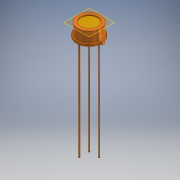
# Autodesk Inventor part: Thorlabs_FDS010
Saved by Autodesk Inventor 2018 (Build 220112000, 112)
## iProperties
Created: 2017-06-15
Part Number: Thorlabs_FDS010
Material: Gold
Document SubType Name: Modeling
Designer: yhlien
Density: 19.3 g/cm^3
Appearance: Metal 1600F Hot
Author: yhlien
Autodesk Inventor part; units mm, degrees
ref_plane "YZ Plane" through (0, 0, 0) normal (1, 0, 0) x (0, 1, 0)
ref_plane "XZ Plane" through (0, 0, 0) normal (0, 1, 0) x (-1, 0, 0)
ref_plane "XY Plane" through (0, 0, 0) normal (0, 0, 1) x (1, 0, 0)
sketch "Sketch1" plane through (0, 0, 0) normal (0, 0, 1) x (1, 0, 0)
  circle A0 centre (0, 0) radius 4.55
  dimension "d0" = 9.1
  constraints: 1 centre point, 1 coincident
  measures "d0" diameter of A0
extrude "Base" add sketch "Sketch1" along normal blind 0.71
sketch "Sketch2" plane through (0, 0, 0.71) normal (0, 0, 1) x (1, 0, 0)
  circle A0 centre (0, 0) radius 4.15
  dimension "d3" = 8.3
  constraints: 1 centre point, 1 coincident
  measures "d3" diameter of A0
extrude "Can: Outer Wall" add sketch "Sketch2" along normal blind 3.9
sketch "Sketch3" plane through (0, 0, 4.61) normal (0, 0, 1) x (1, 0, 0)
  circle A0 centre (0, 0) radius 3.85
  dimension "d6" = 7.7
  constraints: 1 centre point, 1 coincident
  measures "d6" diameter of A0
extrude "Can: Inner Wall" cut sketch "Sketch3" against normal blind 3.9
sketch "Sketch4" plane through (0, 0, 4.61) normal (0, 0, 1) x (1, 0, 0)
  circle A0 centre (0, 0) radius 3.85
  dimension "d9" = 7.7
  constraints: 1 centre point, 1 coincident
  measures "d9" diameter of A0
extrude "Can: Top" add sketch "Sketch4" against normal blind 0.3
sketch "Sketch5" plane through (0, 0, 4.61) normal (0, 0, 1) x (1, 0, 0)
  circle A0 centre (0, 0) radius 3.05
  dimension "d12" = 6.1
  constraints: 1 centre point, 1 coincident
  measures "d12" diameter of A0
extrude "Can: Hole" cut sketch "Sketch5" against normal blind 0.3
ref_plane "Work Plane1" through (0, 0, 4.31) normal (0, 0, 1) x (1, 0, 0)
sketch "Sketch8" plane through (0, 0, 4.31) normal (0, 0, 1) x (1, 0, 0)
  circle A0 centre (0, 0) radius 3.15
  dimension "d16" = 6.3
  constraints: 1 centre point, 1 coincident
  measures "d16" diameter of A0
extrude "Window" add sketch "Sketch8" against normal blind 0.1
sketch "Sketch9" plane through (0, 0, 0) normal (0, 0, -1) x (-1, 0, 0)
  line L0 (0, -0.4) -> (-5.15, -0.4)
  line L1 (-5.15, -0.4) -> (-5.15, 0.4)
  line L2 (-5.15, 0.4) -> (0, 0.4)
  line L3 (0, 0.4) -> (0, -0.4)
  point P0 (0, 0)
  dimension "d19" = 5.15
  dimension "d20" = 0.8
  constraints: 8 end point, 2 parallel, 1 horizontal, 1 perpendicular
  measures "d19" distance of L1.end L2.end
  measures "d20" distance of L0.end L1.end
extrude "Key" add sketch "Sketch9" against normal blind 0.7
sketch "Sketch10" plane through (0, 0, 0) normal (0, 0, -1) x (-1, 0, 0)
  circle A0 centre (-1.803, 1.803) radius 0.25
  point P0 (0, 0)
  dimension "d23" = 0.5
  constraints: 1 centre point
  measures "d23" diameter of A0
extrude "Pin 1" add sketch "Sketch10" along normal blind 38
sketch "Sketch11" plane through (0, 0, 0) normal (0, 0, -1) x (-1, 0, 0)
  circle A0 centre (1.803, 1.803) radius 0.25
  point P0 (0, 0)
  dimension "d26" = 0.5
  constraints: 1 centre point
  measures "d26" diameter of A0
extrude "Pin 2" add sketch "Sketch11" along normal blind 38
sketch "Sketch12" plane through (0, 0, 0) normal (0, 0, -1) x (-1, 0, 0)
  circle A0 centre (1.803, -1.803) radius 0.25
  point P0 (0, 0)
  dimension "d29" = 0.5
  constraints: 1 centre point
  measures "d29" diameter of A0
extrude "Pin 3" add sketch "Sketch12" along normal blind 38
body "Solid1"
